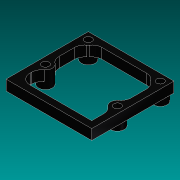
# Autodesk Inventor part: 頭_メインフレーム_1_3
Saved by Autodesk Inventor 2016 (Build 200138000, 138)
## iProperties
Created: 2016-05-11
Part Number: 頭_メインフレーム_1_3
Material: アセタール樹脂、黒
Document SubType Name: Modeling
Designer: hiroaki
Density: 1.425 g/cm^3
Appearance: 滑らか - 黒
Mass: 0.539916 g
Surface Area: 7.97206 cm^2
Volume: 0.378889 cm^3
Author: hiroaki
Autodesk Inventor part; units mm, degrees
ref_plane "YZ Plane" through (0, 0, 0) normal (1, 0, 0) x (0, 1, 0)
ref_plane "XZ Plane" through (0, 0, 0) normal (0, 1, 0) x (-1, 0, 0)
ref_plane "XY Plane" through (0, 0, 0) normal (0, 0, 1) x (1, 0, 0)
sketch "スケッチ1" plane through (0, 0, 0) normal (0, 0, 1) x (1, 0, 0)
  line L0 (-10.5, -6.25) -> (10.5, -6.25) construction
  line L1 (10.5, -6.25) -> (10.5, 6.25) construction
  line L2 (10.5, 6.25) -> (-10.5, 6.25) construction
  line L3 (-10.5, 6.25) -> (-10.5, -6.25) construction
  line L4 (-10.5, -6.25) -> (10.5, 6.25) construction
  line L5 (10.5, -6.25) -> (-10.5, 6.25) construction
  circle A0 centre (-10.5, 6.25) radius 1.05
  circle A1 centre (10.5, 6.25) radius 1.05
  circle A2 centre (10.5, -6.25) radius 1.05
  circle A3 centre (-10.5, -6.25) radius 1.05
  line L6 (-12.5, 8.25) -> (12.5, 8.25)
  line L7 (12.5, 8.25) -> (12.5, -8.25)
  line L8 (12.5, -8.25) -> (-12.5, -8.25)
  line L9 (-12.5, -8.25) -> (-12.5, 8.25)
  line L10 (-8.5, 6.25) -> (8.5, 6.25)
  arc A4 (-10.5, 4.25) -> (-8.5, 6.25) centre (-10.5, 6.25) ccw
  line L11 (-10.5, 4.25) -> (-10.5, -4.25)
  arc A5 (-8.5, -6.25) -> (-10.5, -4.25) centre (-10.5, -6.25) ccw
  arc A6 (8.5, 6.25) -> (10.5, 4.25) centre (10.5, 6.25) ccw
  line L12 (10.5, 4.25) -> (10.5, -4.25)
  arc A7 (10.5, -4.25) -> (8.5, -6.25) centre (10.5, -6.25) ccw
  line L13 (0, 0) -> (0, 8.25) construction
  line L14 (8.5, -6.25) -> (-8.5, -6.25)
  point P0 (0, 0)
  point P1 (0, 0)
  dimension "d0" = 2.1
  dimension "d1" = 21
  dimension "d2" = 12.5
  dimension "d7" = 25
  dimension "d8" = 2
  dimension "d9" = 2
  dimension "d10" = 2
  dimension "d17" = 2
  dimension "d18" = 2
  constraints: 30 end point, 8 centre point, 8 coincident, 8 point on circle, 6 equal radius, 5 midpoint, 4 parallel, 3 collinear, 3 horizontal, 3 vertical, 2 perpendicular, 1 vertical alignment
  measures "d0" diameter of A0
  measures "d1" distance of L1.end L2.end
  measures "d2" distance of L2.end L0.start
  measures "d7" distance of L6.start L6.end
  measures "d8" distance between parallel lines of L6 L10
  measures "d9" distance between parallel lines of L9 L11
  measures "d10" radius of A4
  measures "d17" distance between parallel lines of L7 L12
  measures "d18" distance between parallel lines of L8 L14
extrude "押し出し1" add sketch "スケッチ1" along normal blind 2
fillet "フィレット1" radius 3 8 edges at (-8.5, -6.25, 1) (-10.5, -4.25, 1) (-10.5, 4.25, 1) (-8.5, 6.25, 1) (8.5, -6.25, 1) (10.5, -4.25, 1) (10.5, 4.25, 1) (8.5, 6.25, 1)
sketch "スケッチ2" plane through (0, 0, 0) normal (0, 0, -1) x (-1, 0, 0)
  arc A0 (-8.9, -5.05) -> (-9.3, -4.65) centre (-10.5, -6.25) ccw projected
  circle A1 centre (10.5, -6.25) radius 1.05 projected
  circle A2 centre (-10.5, -6.25) radius 1.05 projected
  circle A3 centre (-10.5, 6.25) radius 1.05 projected
  circle A4 centre (10.5, 6.25) radius 1.05 projected
  circle A5 centre (-10.5, -6.25) radius 2
  circle A6 centre (10.5, -6.25) radius 2
  circle A7 centre (10.5, 6.25) radius 2
  circle A8 centre (-10.5, 6.25) radius 2
  point P0 (0, 0)
  constraints: 4 centre point, 4 coincident, 3 equal radius, 1 concentric
extrude "押し出し2" add sketch "スケッチ2" along normal blind 2
equation "\"d9\" = d8"
equation "\"d17\" = d9"
equation "\"d18\" = d8"
